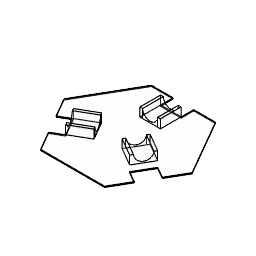
darkviz_base (Autodesk Fusion 360 design; units mm, degrees)
Autodesk Fusion 360 part; units mm, degrees
sketch "Sketch1" plane through (0, 0, 0) normal (0, 1, 0) x (1, 0, 0)
  line L0 (-57.6352, -99.9424) -> (57.735, -99.8847)
  line L1 (115.3702, 0.0576) -> (57.6352, 99.9424)
  line L2 (-57.735, 99.8847) -> (-115.3702, -0.0576)
  line L3 (0, 0) -> (-86.5277, -49.9568)
  line L4 (-77.2777, -65.9783) -> (-57.6679, -54.6435)
  line L5 (-95.7777, -33.9353) -> (-76.1622, -22.6103)
  line L6 (-76.1622, -22.6103) -> (-57.6679, -54.6435)
  line L7 (0, 0) -> (86.5277, -49.9568)
  line L8 (95.7777, -33.9353) -> (76.1566, -22.6201)
  line L9 (77.2777, -65.9783) -> (57.6566, -54.6631)
  line L10 (76.1566, -22.6201) -> (57.6566, -54.6631)
  line L11 (95.7697, -33.9307) -> (115.3702, 0.0576)
  line L12 (57.735, -99.8847) -> (77.2777, -65.9783)
  line L13 (-77.2777, -65.9783) -> (-57.6352, -99.9424)
  line L14 (-95.7777, -33.9353) -> (-115.3702, -0.0576)
  line L15 (18.4501, 99.9228) -> (18.4614, 77.2728)
  line L16 (-18.5499, 99.9043) -> (-18.5386, 77.2543)
  line L17 (-18.5386, 77.2543) -> (18.4614, 77.2728)
  line L18 (18.4501, 99.9228) -> (57.6352, 99.9424)
  line L19 (-57.735, 99.8847) -> (-18.5499, 99.9043)
  dimension "d11" = 18.5
  dimension "d12" = 18.5
  dimension "d13" = 22.65
  dimension "d14" = 22.65
  dimension "d16" = 18.5
  dimension "d17" = 18.5
  dimension "d18" = 22.65
  dimension "d19" = 22.65
  dimension "d22" = 22.65
  dimension "d23" = 22.65
  constraint coincident L3.start L7.start
  constraint perpendicular L8 L11
  constraint coincident L8 L11.start
  constraint perpendicular L15 L18
  constraint perpendicular L16 L19
  measures "d11" distance of L3.end L4.start
  measures "d12" distance of L3.end L5.start
  measures "d13" distance of L4.start L4.end
  measures "d14" distance of L5.start L5.end
  measures "d16" distance of L7.end L8.start
  measures "d17" distance of L7.end L9.start
  measures "d18" distance of L8.start L8.end
  measures "d19" distance of L9.start L9.end
  measures "d22" distance of L15.start L15.end
  measures "d23" distance of L16.start L16.end
extrude "Extrude1" add sketch "Sketch1" along normal blind 2 makes body 1
sketch "Sketch2" plane through (0, 2, 0) normal (0, 1, 0) x (-1, 0, 0)
  line L0 (95.7777, 33.9353) -> (76.1622, 22.6103)
  line L1 (76.1622, 22.6103) -> (57.6679, 54.6435)
  line L2 (57.6679, 54.6435) -> (77.2777, 65.9783)
  line L3 (77.2777, 65.9783) -> (57.6352, 99.9424)
  line L4 (57.6352, 99.9424) -> (-57.735, 99.8847)
  line L5 (-57.735, 99.8847) -> (-77.2777, 65.9783)
  line L6 (-77.2777, 65.9783) -> (-57.6566, 54.6631)
  line L7 (-57.6566, 54.6631) -> (-76.1566, 22.6201)
  line L8 (-76.1566, 22.6201) -> (-95.7697, 33.9307)
  line L9 (-95.7697, 33.9307) -> (-115.3702, -0.0576)
  line L10 (-115.3702, -0.0576) -> (-57.6352, -99.9424)
  line L11 (-57.6352, -99.9424) -> (-18.4501, -99.9228)
  line L12 (-18.4501, -99.9228) -> (-18.4614, -77.2728)
  line L13 (-18.4614, -77.2728) -> (18.5386, -77.2543)
  line L14 (18.5386, -77.2543) -> (18.5499, -99.9043)
  line L15 (18.5499, -99.9043) -> (57.735, -99.8847)
  line L16 (57.735, -99.8847) -> (115.3702, 0.0576)
  line L17 (115.3702, 0.0576) -> (95.7777, 33.9353)
  line L18 (0, 0) -> (-88.4164, 51.0472)
  line L19 (0, 0) -> (79.9444, 46.1559)
  line L20 (-66.9066, 38.6416) -> (-73.7281, 26.8126)
  line L21 (-66.9066, 38.6416) -> (-60.085, 50.4706)
  line L22 (-73.7281, 26.8126) -> (-41.3561, 8.1226)
  line L23 (-60.085, 50.4706) -> (-27.7129, 31.7806)
  line L24 (-41.3561, 8.1226) -> (-27.7129, 31.7806)
  line L25 (-76.1566, 22.6201) -> (-43.7845, 3.9301)
  line L26 (-41.3561, 8.1226) -> (-43.7845, 3.9301)
  line L27 (-57.6566, 54.6631) -> (-25.1484, 35.8945)
  line L28 (-27.7129, 31.7806) -> (-25.1484, 35.8945)
  dimension "d24" = 13.655
  dimension "d25" = 13.655
  dimension "d26" = 37.38
  dimension "d27" = 37.38
  dimension "d28" = 37.38
  constraint coincident L18.start L19.start
  constraint perpendicular L7 L18
  constraint perpendicular L1 L19
  constraint midpoint L7 L20.start
  constraint perpendicular L8 L20
  constraint perpendicular L6 L21
  constraint perpendicular L7 L22
  constraint perpendicular L7 L23
  constraint coincident L7.end L8.start
  constraint perpendicular L7 L25
  constraint coincident L6.end L7.start
  constraint perpendicular L7 L27
  measures "d24" distance of L20.start L20.end
  measures "d25" distance of L20.start L21.end
  measures "d26" distance of L20.end L22.end
  measures "d27" distance of L21.end L23.end
  measures "d28" distance of L7.end L25.end
extrude "Extrude2" add sketch "Sketch2" along normal blind 15.65 separate body contours L18 L20 L22 L24 | L7 L18 L20 L23 L24 | L7 L20 L22 L25 L26 | L7 L23 L27 L28 makes body 2
sketch "Sketch5" plane through (66.9122, 0, 38.6318) normal (0.866025, 0, 0.5) x (0.5, 0, -0.866025)
  line L0 (-18.5113, 0) -> (18.4887, 0)
  line L1 (18.4887, 0) -> (18.4887, 2)
  line L2 (18.4887, 2) -> (18.4887, 17.65)
  line L3 (18.4887, 17.65) -> (-18.5113, 17.65)
  line L4 (-18.5113, 17.65) -> (-18.5113, 2)
  line L5 (-18.5113, 2) -> (-18.5113, 0)
  line L6 (0, 2) -> (13.655, 2)
  line L7 (-0.0113, -9.66) -> (-13.6663, -9.66)
  line L8 (13.655, 2) -> (13.655, 29.31)
  line L9 (-13.6663, -9.66) -> (-13.6663, 17.65)
  line L10 (18.4887, 2) -> (-18.5113, 2)
  line L11 (-18.5113, 2) -> (18.4887, 2)
  dimension "d32" = 13.655
  dimension "d33" = 13.655
  constraint coincident L3 L9.end
  constraint perpendicular L3 L9
  measures "d32" distance of L6.start L6.end
  measures "d33" distance of L7.start L7.end
sketch "Sketch6" plane through (66.9122, 0, 38.6318) normal (0.866025, 0, 0.5) x (0.5, 0, -0.866025)
  line L0 (0, 18.3) -> (18.5, 18.3)
  line L1 (0, 18.3) -> (-18.5, 18.3)
  arc A0 (-13.655, 18.3) -> (13.655, 18.3) centre (0, 18.3) ccw
  dimension "d34" = 27.31
  constraint coincident L0.start L1.start
  constraint horizontal L0
  constraint horizontal L1
  constraint coincident L0 A0.end
  constraint coincident L1 A0.start
  measures "d34" diameter of A0
extrude "Extrude3" cut sketch "Sketch6" against normal blind 42 bodies 1 2
sketch "Sketch7" plane through (0, 2, 0) normal (0, 1, 0) x (-1, 0, 0)
  line L0 (-76.1566, 22.6201) -> (-95.7697, 33.9307)
  line L1 (-95.7697, 33.9307) -> (-115.3702, -0.0576)
  line L2 (-115.3702, -0.0576) -> (-57.6352, -99.9424)
  line L3 (-57.6352, -99.9424) -> (-18.4501, -99.9228)
  line L4 (-18.4501, -99.9228) -> (-18.4614, -77.2728)
  line L5 (-18.4614, -77.2728) -> (18.5386, -77.2543)
  line L6 (18.5386, -77.2543) -> (18.5499, -99.9043)
  line L7 (18.5499, -99.9043) -> (57.735, -99.8847)
  line L8 (57.735, -99.8847) -> (115.3702, 0.0576)
  line L9 (115.3702, 0.0576) -> (95.7777, 33.9353)
  line L10 (95.7777, 33.9353) -> (76.1622, 22.6103)
  line L11 (76.1622, 22.6103) -> (57.6679, 54.6435)
  line L12 (57.6679, 54.6435) -> (77.2777, 65.9783)
  line L13 (77.2777, 65.9783) -> (57.6352, 99.9424)
  line L14 (57.6352, 99.9424) -> (-57.735, 99.8847)
  line L15 (-57.735, 99.8847) -> (-77.2777, 65.9783)
  line L16 (-77.2777, 65.9783) -> (-57.6566, 54.6631)
  line L17 (-57.6566, 54.6631) -> (-76.1566, 22.6201)
pattern_circular "C-Pattern1" count 3 over 360 about axis through (0, 1.75, 0) along (0, 1, 0) of bodies 2 makes body 3 at (-11.6029, 11.1006, -64.8016) makes body 4 at (-50.3184, 11.1006, 42.4492)
copy_body "CutPasteBodies1" bodies 4 removing the originals makes body 5
move_body "Move1" bodies 2 to x (1, 0, 0) y (0, 1, 0) z (0, 0, 1) at (0, 10.4, 0)
